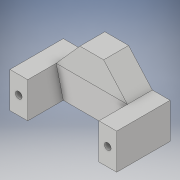
# Autodesk Inventor part: sliding piece for grabber
Saved by Autodesk Inventor 2019 (Build 230136000, 136)
## iProperties
Created: 2019-11-09
Part Number: sliding piece for grabber
Material: Generic
Document SubType Name: Modeling
Designer: User
Density: 1 g/cm^3
Appearance: Default
Author: User
Autodesk Inventor part; units mm, degrees
ref_plane "YZ Plane" through (0, 0, 0) normal (1, 0, 0) x (0, 1, 0)
ref_plane "XZ Plane" through (0, 0, 0) normal (0, 1, 0) x (-1, 0, 0)
ref_plane "XY Plane" through (0, 0, 0) normal (0, 0, 1) x (1, 0, 0)
sketch "Sketch1" plane through (0, 0, 0) normal (0, 1, 0) x (-1, 0, 0)
  line L0 (0, 0) -> (12.7, 0)
  line L1 (12.7, 0) -> (12.7, 38.1)
  line L2 (12.7, 38.1) -> (0, 38.1)
  line L3 (0, 38.1) -> (0, 0)
  line L4 (12.7, 0) -> (63.5, 0)
  line L5 (63.5, 0) -> (63.5, 12.7)
  line L6 (63.5, 12.7) -> (12.7, 12.7)
  line L7 (12.7, 12.7) -> (12.7, 0)
  line L8 (63.5, 0) -> (76.2, 0)
  line L9 (76.2, 0) -> (76.2, 38.1)
  line L10 (76.2, 38.1) -> (63.5, 38.1)
  line L11 (63.5, 38.1) -> (63.5, 0)
  dimension "d0" = 38.1
  dimension "d1" = 38.1
  dimension "d2" = 12.7
  dimension "d3" = 12.7
  dimension "d5" = 50.8
  dimension "d6" = 12.7
  constraints: 24 end point, 6 parallel, 3 horizontal, 3 perpendicular
  measures "d0" distance of L2.end L0.start
  measures "d1" distance of L8.end L9.end
  measures "d2" distance of L0.start L0.end
  measures "d3" distance of L4.end L8.end
  measures "d5" distance of L5.end L6.end
  measures "d6" distance between parallel lines of L6 L4
extrude "Extrusion1" add sketch "Sketch1" along normal blind 25.4
sketch "Sketch2" plane through (-63.5, 0, 38.1) normal (1, 0, 0) x (0, 0, -1)
  line L0 (25.4, 0) -> (25.4, 25.4) projected
  line L1 (25.4, 0) -> (20.32, 25.4)
  line L2 (0, 25.4) -> (25.4, 25.4) projected
  point P0 (38.1, 0)
  dimension "d9" = 5.08
  constraints: 2 end point, 1 point on line
  measures "d9" distance of L0.end L1.end
extrude "Extrusion2" add sketch "Sketch2" along normal blind 50.8
sketch "Sketch3" plane through (-76.2, 0, 38.1) normal (0, 0, 1) x (1, 0, 0)
  line L0 (0, 25.4) -> (12.7, 25.4) projected
  line L1 (0, 0) -> (0, 25.4) projected
  line L2 (63.5, 25.4) -> (76.2, 25.4) projected
  line L3 (76.2, 0) -> (76.2, 25.4) projected
  point P0 (6.35, 12.7)
  point P1 (69.85, 12.7)
  dimension "d12" = 12.7
  dimension "d13" = 25.4
  dimension "d14" = 6.35
  dimension "d15" = 12.7
  dimension "d16" = 12.7
  dimension "d17" = 25.4
  dimension "d18" = 12.7
  dimension "d19" = 6.35
  measures "d12" distance of L0.start L0.end
  measures "d13" distance of L1.start L0.start
  measures "d14" distance from line of L1 point (6.35, 12.7)
  measures "d15" distance from line of point (6.35, 12.7) L0
  measures "d16" distance of L2.start L2.end
  measures "d17" distance of L3.start L2.end
  measures "d18" distance from line of point (69.85, 12.7) L2
  measures "d19" distance from line of L3 point (69.85, 12.7)
hole "Hole1" at (-69.85, 12.7, 38.1) at (-6.35, 12.7, 38.1) direction (0, 0, -1) diameter 4.7625 end through all
sketch "Sketch4" plane through (0, 25.4, 0) normal (0, 1, 0) x (1, 0, 0)
  line L0 (0, 0) -> (-76.2, 0) projected
  line L1 (0, -38.1) -> (0, 0) projected
  line L2 (-12.7, -17.78) -> (-12.7, -38.1) projected
  point P0 (-38.1, -8.89)
  dimension "d27" = 38.1
  dimension "d28" = 20.32
  dimension "d29" = 76.2
  dimension "d30" = 38.1
  dimension "d31" = 8.89
  measures "d27" distance of L1.start L0.start
  measures "d28" distance of L2.start L2.end
  measures "d29" distance of L0.start L0.end
  measures "d30" distance from line of L1 point (-38.1, -8.89)
  measures "d31" distance from line of L0 point (-38.1, -8.89)
hole "Hole2" at (-38.1, 25.4, 8.89) direction (0, -1, 0) diameter 2.6416 end through all thread size "6-32 UNC" class "2B" standard "ANSI Unified Screw Threads"
sketch "Sketch5" plane through (0, 25.4, 0) normal (0, 1, 0) x (1, 0, 0)
  line L0 (-63.5, -17.78) -> (-12.7, -17.78) projected
  line L1 (0, 0) -> (-76.2, 0) projected
  line L2 (-63.5, -17.78) -> (-12.7, -17.78)
  line L3 (-12.7, -17.78) -> (-12.7, 0)
  line L4 (-12.7, 0) -> (-63.5, 0)
  line L5 (-63.5, 0) -> (-63.5, -17.78)
  line L6 (-12.7, -38.1) -> (0, -38.1) projected
  line L7 (0, -38.1) -> (0, 0) projected
  dimension "d39" = 12.7
  dimension "d40" = 12.7
  constraints: 8 end point, 2 parallel, 1 horizontal, 1 perpendicular, 1 point on line
  measures "d39" distance of L6.start L6.end
  measures "d40" distance between parallel lines of L7 L3
extrude "Extrusion3" add sketch "Sketch5" along normal blind 19.05
sketch "Sketch6" plane through (-63.5, 25.4, 17.78) normal (0, 0, 1) x (1, 0, 0)
  line L0 (0, 0) -> (50.8, 0) projected
  line L1 (0, 0) -> (16.9333, 19.05)
  line L2 (50.8, 19.05) -> (0, 19.05) projected
  line L3 (63.5, 0) -> (50.8, 0) projected
  line L4 (50.8, 0) -> (33.8667, 19.05)
  line L5 (0, 0) -> (0, 19.05) projected
  line L6 (0, 0) -> (50.8, 0) projected
  line L7 (50.8, 0) -> (50.8, 19.05) projected
  line L8 (0, 19.05) -> (50.8, 19.05) projected
  line L9 (0, 0) -> (0, 19.05) projected
  point P0 (63.5, -25.4)
  dimension "d43" = 50.8
  dimension "d44" = 16.9333
  dimension "d45" = 16.9333
  constraints: 4 end point, 2 point on line
  measures "d43" distance of L2.start L2.end
  measures "d44" distance of L1.end L2.end
  measures "d45" distance of L2.start L4.end
extrude "Extrusion4" cut sketch "Sketch6" against normal blind 19.05 contours L5 L2 L1 | L4 L2 L7
equation "\"d1\" = d0"
equation "\"d3\" = d2"
equation "\"d14\" = 0.5 * d12"
equation "\"d15\" = 0.5 * d13"
equation "\"d18\" = 0.5 * d17"
equation "\"d19\" = 0.5 * d16"
equation "\"d30\" = 0.5 * d29"
equation "\"d31\" = -0.5 * d28 + 0.5 * d27"
equation "\"d40\" = d39"
equation "\"d44\" = 0.333333 * d43"
equation "\"d45\" = 0.333333 * d43"
body "Solid1"
